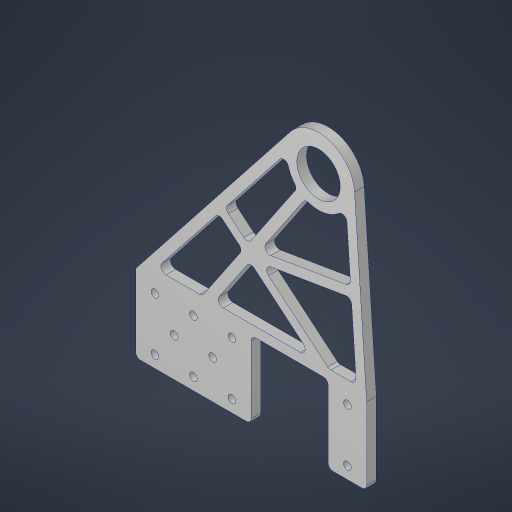
# Autodesk Inventor part: CL3-004
Saved by Autodesk Inventor 2023.4 (Build 274418000, 418)
## iProperties
Created: 2025-01-28
Part Number: CL3-004
Material: Aluminum 6061
Document SubType Name: Modeling
Designer: slick
Density: 2.7 g/cm^3
Appearance: Aluminum - Flat
Mass: 311.171 g
Surface Area: 423.623 cm^2
Volume: 115.249 cm^3
Author: slick
Autodesk Inventor part; units mm, degrees
ref_plane "YZ Plane" through (0, 0, 0) normal (1, 0, 0) x (0, 1, 0)
ref_plane "XZ Plane" through (0, 0, 0) normal (0, 1, 0) x (-1, 0, 0)
ref_plane "XY Plane" through (0, 0, 0) normal (0, 0, 1) x (1, 0, 0)
sketch "Sketch1" plane through (0, 0, 0) normal (0, 0, 1) x (1, 0, 0)
  line L0 (-76.2, 25.4) -> (76.2, 25.4) construction
  line L1 (76.2, 25.4) -> (76.2, -25.4) construction
  line L2 (76.2, -25.4) -> (-76.2, -25.4) construction
  line L3 (-76.2, -25.4) -> (-76.2, 25.4) construction
  line L4 (-76.2, 25.4) -> (76.2, -25.4) construction
  line L5 (76.2, 25.4) -> (-76.2, -25.4) construction
  line L6 (63.5, 17.4625) -> (63.5, -17.4625) construction
  line L7 (9.525, 15.875) -> (41.275, 15.875) construction
  line L8 (41.275, 15.875) -> (41.275, -15.875) construction
  line L9 (41.275, -15.875) -> (9.525, -15.875) construction
  line L10 (9.525, -15.875) -> (9.525, 15.875) construction
  line L11 (9.525, 15.875) -> (41.275, -15.875) construction
  line L12 (41.275, 15.875) -> (9.525, -15.875) construction
  line L13 (76.2, 101.6) -> (187.452, 101.6) construction
  line L14 (187.452, 101.6) -> (187.452, -25.4) construction
  line L15 (187.452, -25.4) -> (76.2, -25.4) construction
  line L16 (76.2, -25.4) -> (76.2, 101.6) construction
  line L17 (76.2, 101.6) -> (187.452, -25.4) construction
  line L18 (187.452, 101.6) -> (76.2, -25.4) construction
  point P0 (0, 0)
  point P1 (63.5, 0)
  point P2 (25.4, 0)
  point P3 (50.8, 0)
  point P4 (0, 0)
  point P5 (9.525, 0)
  point P6 (-12.7, 17.4625)
  point P7 (-12.7, -17.4625)
  point P8 (-25.4, 0)
  point P9 (-38.1, 17.4625)
  point P10 (-38.1, -17.4625)
  point P11 (-50.8, 0)
  point P12 (-63.5, 17.4625)
  point P13 (-63.5, -17.4625)
  point P14 (131.826, 38.1)
  dimension "d0" = 152.4
  dimension "d1" = 50.8
  dimension "d2" = 34.925
  dimension "d3" = 12.7
  dimension "d4" = 31.75
  dimension "d5" = 31.75
  dimension "d6" = 34.925
  dimension "d7" = 25.4
  dimension "d8" = 9.525
  dimension "d9" = 12.7
  dimension "d10" = 12.7
  dimension "d11" = 12.7
  dimension "d12" = 12.7
  dimension "d13" = 12.7
  dimension "d14" = 111.252
  dimension "d15" = 127
  dimension "d16" = 76.2
  constraints: 38 end point, 11 horizontal alignment, 8 midpoint, 6 parallel, 4 vertical alignment, 3 horizontal, 3 perpendicular, 2 coincident, 1 vertical
  measures "d0" distance of L1.end L2.end
  measures "d1" distance of L0.end L1.end
  measures "d2" distance of L6.end L6.start
  measures "d3" distance from line of L1 L6.start
  measures "d4" distance of L8.end L9.end
  measures "d5" distance of L7.end L8.end
  measures "d6" distance between parallel lines of L1 L8
  measures "d7" distance from line of L1 point (50.8, 0)
  measures "d8" distance of point (9.525, 0) point (0, 0)
  measures "d9" horizontal distance of point (0, 0) point (-12.7, 17.463)
  measures "d10" horizontal distance of point (-38.1, 17.463) point (-25.4, 0)
  measures "d11" horizontal distance of point (-38.1, -17.463) point (-50.8, 0)
  measures "d12" horizontal distance of point (-12.7, -17.463) point (-25.4, 0)
  measures "d13" horizontal distance of point (-63.5, 17.463) point (-50.8, 0)
  measures "d14" distance of L14.end L15.end
  measures "d15" distance of L13.end L14.end
  measures "d16" distance between parallel lines of L13 L0
sketch "Sketch2" plane through (0, 0, 0) normal (0, 0, 1) x (1, 0, 0)
  line L0 (63.5, 17.4625) -> (63.5, -17.4625) construction
  line L1 (76.2, 25.4) -> (76.2, -25.4) construction
  line L2 (76.2, -25.4) -> (76.2, 101.6) construction
  line L3 (187.452, -25.4) -> (76.2, -25.4) construction
  line L4 (187.452, 101.6) -> (187.452, -25.4) construction
  line L5 (76.2, 101.6) -> (187.452, -25.4) construction
  line L6 (187.452, 101.6) -> (76.2, -25.4) construction
  line L7 (76.2, 101.6) -> (187.452, 101.6) construction
  line L8 (9.525, 15.875) -> (41.275, 15.875) construction
  line L9 (41.275, 15.875) -> (41.275, -15.875) construction
  line L10 (41.275, -15.875) -> (9.525, -15.875) construction
  line L11 (9.525, -15.875) -> (9.525, 15.875) construction
  line L12 (9.525, 15.875) -> (41.275, -15.875) construction
  line L13 (41.275, 15.875) -> (9.525, -15.875) construction
  line L14 (-76.2, 25.4) -> (76.2, 25.4) construction
  line L15 (76.2, -25.4) -> (-76.2, -25.4) construction
  line L16 (-76.2, 25.4) -> (76.2, -25.4) construction
  line L17 (76.2, 25.4) -> (-76.2, -25.4) construction
  line L18 (-76.2, -25.4) -> (-76.2, 25.4) construction
  line L19 (0, 25.4) -> (0, -25.4)
  line L20 (0, -25.4) -> (-76.2, -25.4)
  line L21 (-76.2, -25.4) -> (-76.2, 25.4)
  line L22 (-76.2, 25.4) -> (25.7652, 154.4619)
  circle A0 centre (44.45, 139.7) radius 14.2875
  circle A1 centre (44.45, 139.7) radius 23.8125 construction
  line L23 (68.2061, 141.338) -> (76.2, 25.4)
  line L24 (76.2, 25.4) -> (76.2, -25.4)
  line L25 (76.2, -25.4) -> (50.8, -25.4)
  line L26 (50.8, -25.4) -> (50.8, 25.4)
  line L27 (50.8, 25.4) -> (0, 25.4)
  arc A2 (68.2061, 141.338) -> (25.7652, 154.4619) centre (44.45, 139.7) ccw
  point P0 (0, 0)
  point P1 (63.5, 0)
  point P2 (131.826, 38.1)
  point P3 (9.525, 0)
  point P4 (0, 0)
  point P5 (25.4, 0)
  point P6 (-63.5, -17.4625)
  point P7 (-63.5, 17.4625)
  point P8 (-50.8, 0)
  point P9 (-38.1, -17.4625)
  point P10 (-38.1, 17.4625)
  point P11 (-25.4, 0)
  point P12 (-12.7, -17.4625)
  point P13 (-12.7, 17.4625)
  point P14 (0, 0)
  point P15 (50.8, 0)
  point P16 (0, 0)
  dimension "d17" = 28.575
  dimension "d18" = 9.525
  dimension "d20" = 9.525
  dimension "d21" = 9.525
  dimension "d31" = 165.1
  dimension "d32" = 19.05
  constraints: 18 end point, 4 point on circle, 3 centre point, 3 coincident, 3 midpoint, 2 collinear, 2 point on line, 2 tangent, 1 perpendicular
  measures "d17" diameter of A0
  measures "d18" radial gap between concentric circles of A0 A1
  measures "d20" distance between parallel lines of L11 L19
  measures "d21" distance between parallel lines of L26 L9
  measures "d31" distance from line of L15 A0.centre
  measures "d32" horizontal distance of point (63.5, 17.463) A0.centre
extrude "Extrusion1" add sketch "Sketch2" along normal blind 6.35
hole "Hole1" at (76.2, 101.6, 0) at (131.826, 38.1, 0) at (187.452, -25.4, 0) at (9.525, 0, 0) at (9.525, 15.875, 0) at (41.275, -15.875, 0) at (41.275, 15.875, 0) at (9.525, -15.875, 0) at (25.4, 0, 0) at (-63.5, -17.4625, 0) at (-63.5, 17.4625, 0) at (-50.8, 0, 0) at (-38.1, -17.4625, 0) at (-38.1, 17.4625, 0) at (-25.4, 0, 0) at (-12.7, -17.4625, 0) at (-12.7, 17.4625, 0) at (63.5, 17.4625, 0) at (63.5, -17.4625, 0) direction (0, 0, 1) diameter 5.1054 end through all clearance for "Flat Head Machine Screw (82)" size "#10" standard "Ansi Unified Screw Threads"
fillet "Fillet1" radius 3.175 7 edges at (50.8, 25.4, 3.175) (0, 25.4, 3.175) (0, -25.4, 3.175) (50.8, -25.4, 3.175) (76.2, -25.4, 3.175) (-76.2, -25.4, 3.175) (-76.2, 25.4, 3.175)
sketch "Sketch3" plane through (0, 0, 6.35) normal (0, 0, 1) x (1, 0, 0)
  circle A0 centre (63.5, 17.4625) radius 2.5527 construction
  circle A1 centre (-12.7, -17.4625) radius 2.5527 construction
  circle A2 centre (-38.1, 17.4625) radius 2.5527 construction
  circle A3 centre (-50.8, 0) radius 2.5527 construction
  circle A4 centre (-63.5, -17.4625) radius 2.5527 construction
  circle A5 centre (-63.5, 17.4625) radius 2.5527 construction
  circle A6 centre (-38.1, -17.4625) radius 2.5527 construction
  circle A7 centre (-25.4, 0) radius 2.5527 construction
  circle A8 centre (-12.7, 17.4625) radius 2.5527 construction
  circle A9 centre (63.5, -17.4625) radius 2.5527 construction
  circle A10 centre (44.45, 139.7) radius 14.2875 construction
  arc A11 (68.2061, 141.338) -> (25.7652, 154.4619) centre (44.45, 139.7) ccw construction
  line L0 (68.2061, 141.338) -> (76.2, 25.4) construction
  line L1 (76.2, 25.4) -> (76.2, -22.225) construction
  arc A12 (73.025, -25.4) -> (76.2, -22.225) centre (73.025, -22.225) ccw construction
  line L2 (73.025, -25.4) -> (53.975, -25.4) construction
  arc A13 (50.8, -22.225) -> (53.975, -25.4) centre (53.975, -22.225) ccw construction
  line L3 (50.8, -22.225) -> (50.8, 22.225) construction
  arc A14 (50.8, 22.225) -> (47.625, 25.4) centre (47.625, 22.225) ccw construction
  line L4 (47.625, 25.4) -> (3.175, 25.4) construction
  arc A15 (3.175, 25.4) -> (0, 22.225) centre (3.175, 22.225) ccw construction
  line L5 (0, 22.225) -> (0, -22.225) construction
  arc A16 (-3.175, -25.4) -> (0, -22.225) centre (-3.175, -22.225) ccw construction
  line L6 (-3.175, -25.4) -> (-73.025, -25.4) construction
  arc A17 (-76.2, -22.225) -> (-73.025, -25.4) centre (-73.025, -22.225) ccw construction
  line L7 (-76.2, -22.225) -> (-76.2, 24.2971) construction
  arc A18 (-75.5163, 26.2654) -> (-76.2, 24.2971) centre (-73.025, 24.2971) ccw construction
  line L8 (-75.5163, 26.2654) -> (25.7652, 154.4619) construction
  circle A19 centre (44.45, 139.7) radius 20.6375 construction
  line L9 (69.85, 25.1813) -> (61.8711, 140.9012) construction
  arc A20 (61.8711, 140.9012) -> (30.7478, 150.5254) centre (44.45, 139.7) ccw construction
  line L10 (30.7478, 150.5254) -> (-69.85, 23.1943) construction
  line L11 (-69.85, 23.1943) -> (-69.85, -19.05) construction
  line L12 (-69.85, -19.05) -> (-6.35, -19.05) construction
  line L13 (-6.35, -19.05) -> (-6.35, 22.225) construction
  arc A21 (3.175, 31.75) -> (-6.35, 22.225) centre (3.175, 22.225) ccw construction
  line L14 (3.175, 31.75) -> (47.625, 31.75) construction
  arc A22 (57.15, 22.225) -> (47.625, 31.75) centre (47.625, 22.225) ccw construction
  line L15 (57.15, 22.225) -> (57.15, -19.05) construction
  line L16 (57.15, -19.05) -> (69.85, -19.05) construction
  line L17 (69.85, -19.05) -> (69.85, 25.1813) construction
  line L18 (3.175, 31.75) -> (-63.0905, 31.75) construction
  line L19 (47.625, 31.75) -> (69.3971, 31.75) construction
  circle A23 centre (-38.1, 17.4625) radius 2.5527 construction
  line L20 (-38.1, 17.4625) -> (44.45, 139.7) construction
  circle A24 centre (63.5, 17.4625) radius 2.5527 construction
  line L21 (63.5, 17.4625) -> (-19.5511, 86.8598) construction
  line L22 (65.8606, 83.0413) -> (-1.4492, 71.7339) construction
  line L23 (65.6411, 86.2239) -> (5.3247, 76.0913) construction
  line L24 (-24.6201, 31.75) -> (58.4936, 154.8223) construction
  line L25 (-32.2825, 31.75) -> (30.4064, 124.5777) construction
  line L26 (41.4499, 31.75) -> (-21.5201, 84.3676) construction
  line L27 (51.353, 31.75) -> (-17.5821, 89.3521) construction
  line L28 (66.08, 79.8586) -> (5.8815, 69.7459) construction
  line L29 (65.6411, 86.2239) -> (5.3247, 76.0913)
  line L30 (5.3247, 76.0913) -> (35.6688, 121.0239)
  line L31 (65.6411, 86.2239) -> (62.6277, 129.9287)
  arc A25 (35.6688, 121.0239) -> (62.6277, 129.9287) centre (44.45, 139.7) ccw
  line L32 (66.08, 79.8586) -> (5.8815, 69.7459)
  line L33 (5.8815, 69.7459) -> (51.353, 31.75)
  line L34 (51.353, 31.75) -> (69.3971, 31.75)
  line L35 (69.3971, 31.75) -> (66.08, 79.8586)
  line L36 (41.4499, 31.75) -> (-24.6201, 31.75)
  line L37 (-24.6201, 31.75) -> (-0.7863, 67.0424)
  line L38 (-0.7863, 67.0424) -> (41.4499, 31.75)
  line L39 (30.4064, 124.5777) -> (-2.1121, 76.4254)
  line L40 (-2.1121, 76.4254) -> (-17.5821, 89.3521)
  line L41 (-17.5821, 89.3521) -> (23.9296, 141.8953)
  arc A26 (23.9296, 141.8953) -> (30.4064, 124.5777) centre (44.45, 139.7) ccw
  line L42 (-21.5201, 84.3676) -> (-5.6845, 71.1354)
  line L43 (-5.6845, 71.1354) -> (-32.2825, 31.75)
  line L44 (-32.2825, 31.75) -> (-63.0905, 31.75)
  line L45 (-63.0905, 31.75) -> (-21.5201, 84.3676)
  point P0 (0, 0)
  dimension "d34" = 6.35
  dimension "d35" = 6.35
  dimension "d36" = 3.175
  dimension "d37" = 3.175
  dimension "d38" = 3.175
  dimension "d39" = 3.175
  dimension "d40" = 3.175
  dimension "d41" = 3.175
  constraints: 70 end point, 34 point on line, 15 point on circle, 6 centre point, 6 parallel, 2 coincident, 2 horizontal, 2 tangent, 33 other
  measures "d34" radial gap between concentric circles of A10 A19
  measures "d36" distance between parallel lines of L22 L23
  measures "d37" distance between parallel lines of L20 L24
  measures "d38" distance between parallel lines of L20 L25
  measures "d39" distance between parallel lines of L21 L26
  measures "d40" distance between parallel lines of L21 L27
  measures "d41" distance between parallel lines of L22 L28
extrude "Extrusion2" cut sketch "Sketch3" against normal through all
fillet "Fillet2" radius 3.302 19 edges at (-21.5201, 84.3676, 3.175) (-63.0905, 31.75, 3.175) (-32.2825, 31.75, 3.175) (-5.6845, 71.1354, 3.175) (-0.7863, 67.0424, 3.175) (-24.6201, 31.75, 3.175) (41.4499, 31.75, 3.175) (30.4064, 124.5777, 3.175) (23.9296, 141.8953, 3.175) (-17.5821, 89.3521, 3.175) (-2.1121, 76.4254, 3.175) (66.08, 79.8586, 3.175) (5.8815, 69.7459, 3.175) (51.353, 31.75, 3.175) (69.3971, 31.75, 3.175) (65.6411, 86.2239, 3.175) (62.6277, 129.9287, 3.175) (35.6688, 121.0239, 3.175) (5.3247, 76.0913, 3.175)
equation "\"d34\" = off"
equation "\"d35\" = off"
equation "\"d36\" = 0.5 * off"
equation "\"d37\" = 0.5 * off"
equation "\"d38\" = 0.5 * off"
equation "\"d39\" = 0.5 * off"
equation "\"d40\" = 0.5 * off"
equation "\"d41\" = 0.5 * off"
equation "\"off\" = 6.35"
body "Solid1"
